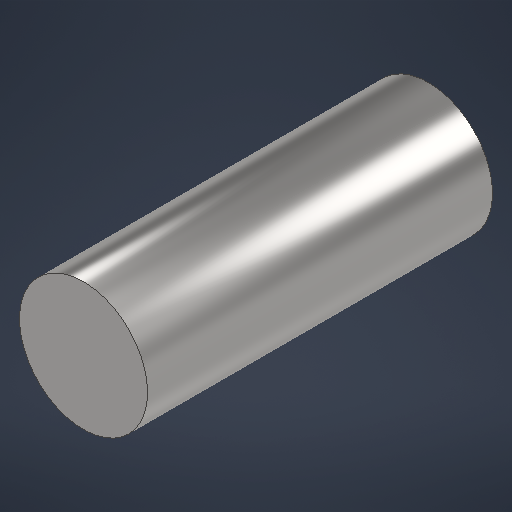
# Autodesk Inventor part: csap1
Saved by Autodesk Inventor 2026.1 (Build 301233000, 233)
## iProperties
Created: 2026-04-13
Part Number: csap1
Material: Steel, Alloy
Document SubType Name: Modeling
Designer: petruska.milan
Density: 7.73 g/cm^3
Appearance: Semi-Polished
Author: petruska.milan
Autodesk Inventor part; units mm, degrees
ref_plane "YZ Plane" through (0, 0, 0) normal (1, 0, 0) x (0, 1, 0)
ref_plane "XZ Plane" through (0, 0, 0) normal (0, 1, 0) x (-1, 0, 0)
ref_plane "XY Plane" through (0, 0, 0) normal (0, 0, 1) x (1, 0, 0)
sketch "Sketch1" plane through (0, 0, 0) normal (0, 1, 0) x (-1, 0, 0)
  line L0 (0, 0) -> (0, -80)
  line L1 (0, -80) -> (-15, -80)
  line L2 (-15, -80) -> (-15, -50)
  line L3 (-15, -50) -> (-12.5, -50)
  line L4 (-12.5, -50) -> (-12.5, -45)
  line L5 (-12.5, -45) -> (-9, -30)
  line L6 (-9, -30) -> (-9, -20)
  line L7 (-9, -20) -> (-6, -20)
  line L8 (-6, -20) -> (-6, 0)
  line L9 (-6, 0) -> (0, 0)
  dimension "d0" = 80
  dimension "d1" = 30
  dimension "d2" = 30
  dimension "d3" = 25
  dimension "d4" = 10
  dimension "d5" = 20
  dimension "d6" = 12
  dimension "d7" = 18
  dimension "d8" = 15
  constraints: 20 end point, 6 perpendicular, 1 horizontal, 1 parallel, 1 vertical
  measures "d0" distance of L0.start L0.end
  measures "d1" distance of L1.end L2.end
  measures "d2" diameter of L2 L0
  measures "d3" diameter of L4 L0
  measures "d4" distance of L5.end L6.end
  measures "d5" distance of L7.end L8.end
  measures "d6" diameter of L8 L0
  measures "d7" diameter of L6 L0
  measures "d8" vertical distance of L4.end L5.end
revolve "Revolution1" add sketch "Sketch1" angle 360 about axis through (0, 0, 0) along (0, 0, -1)
sketch "Sketch2" plane through (0, 0, 0) normal (0, 1, 0) x (-1, 0, 0)
  line L0 (9, -20) -> (9, -30) projected
  line L1 (9, -22) -> (7.5, -22)
  line L2 (7.5, -22) -> (7.5, -24)
  line L3 (7.5, -24) -> (9, -24)
  line L4 (9, -24) -> (9, -22)
  line L5 (0, 0) -> (0, 6.2999)
  line L6 (-9, -20) -> (9, -20) projected
  dimension "d10" = 15
  dimension "d11" = 2
  dimension "d12" = 2
  constraints: 10 end point, 2 parallel, 1 horizontal, 1 perpendicular, 1 point on line, 1 vertical
  measures "d10" diameter of L2 L5
  measures "d11" distance of L1.end L2.end
  measures "d12" distance between parallel lines of L6 L1
revolve "Revolution2" cut sketch "Sketch2" angle 360 about axis through (0, 0, 0) along (0, 0, 1)
pattern_linear "Rectangular Pattern1" count 2 spacing 4 along (0, 0, -1) of "Revolution2"
thread "Thread1" size "M12x1" class "6g" standard "ISO Metric profile" length 15
chamfer "Chamfer1" distance 1 angle 45 1 edges at (-6, 0, 0)
sketch "Sketch3" plane through (0, 0, 0) normal (0, 1, 0) x (-1, 0, 0)
  line L0 (-15, -80) -> (15, -80) projected
  line L1 (-15, -80) -> (0, -80)
  line L2 (0, -80) -> (0, 0.8)
  line L3 (0, 0.8) -> (-15, 0.8)
  line L4 (-15, 0.8) -> (-15, -80)
  line L5 (-15, -50) -> (-15, -80) projected
  line L6 (-5, 0) -> (5, 0) projected
  point P0 (0, 0)
  dimension "d22" = 0.8
  dimension "d23" = 30
  constraints: 8 end point, 2 parallel, 1 horizontal, 1 perpendicular
  measures "d22" distance between parallel lines of L3 L6
  measures "d23" diameter of L4 L2
revolve "Revolution3" add sketch "Sketch3" angle 360 about axis through (0, 0, -80) along (0, 0, 1) separate body
